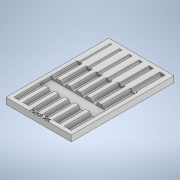
# Autodesk Inventor part: punchTray
Saved by Autodesk Inventor 2020.2 (Build 242310000, 310)
## iProperties
Created: 2019-12-07
Part Number: punchTray
Material: Generic
Document SubType Name: Modeling
Designer: robst
Density: 1 g/cm^3
Appearance: Default
Author: robst
Autodesk Inventor part; units mm, degrees
(part 1 of 2)
ref_plane "YZ Plane" through (0, 0, 0) normal (1, 0, 0) x (0, 1, 0)
ref_plane "XZ Plane" through (0, 0, 0) normal (0, 1, 0) x (-1, 0, 0)
ref_plane "XY Plane" through (0, 0, 0) normal (0, 0, 1) x (1, 0, 0)
sketch "Sketch3" plane through (0, 0, 0) normal (0, 0, 1) x (1, 0, 0)
  line L0 (-52.4636, -4.8895) -> (52.4636, -4.8895)
  line L1 (52.4636, -4.8895) -> (52.4636, 4.8895)
  line L2 (52.4636, 4.8895) -> (-52.4636, 4.8895)
  line L3 (-52.4636, 4.8895) -> (-52.4636, -4.8895)
  line L4 (-52.4636, -4.8895) -> (52.4636, 4.8895) construction
  line L5 (52.4636, -4.8895) -> (-52.4636, 4.8895) construction
  line L6 (46.1136, 4.8895) -> (43.2173, -0.127)
  line L7 (43.2173, -0.127) -> (37.4248, -0.127)
  line L8 (37.4248, -0.127) -> (34.5285, 4.8895)
  line L9 (34.5285, 4.8895) -> (37.4248, 9.906)
  line L10 (37.4248, 9.906) -> (43.2173, 9.906)
  line L11 (43.2173, 9.906) -> (46.1136, 4.8895)
  line L12 (28.1785, 4.8895) -> (25.2822, -0.127)
  line L13 (25.2822, -0.127) -> (19.4897, -0.127)
  line L14 (19.4897, -0.127) -> (16.5934, 4.8895)
  line L15 (16.5934, 4.8895) -> (19.4897, 9.906)
  line L16 (19.4897, 9.906) -> (25.2822, 9.906)
  line L17 (25.2822, 9.906) -> (28.1785, 4.8895)
  line L18 (0, 0) -> (0, 4.8895) construction
  line L19 (10.2434, 4.8895) -> (7.787, 0.635)
  line L20 (7.787, 0.635) -> (2.8744, 0.635)
  line L21 (2.8744, 0.635) -> (0.418, 4.8895)
  line L22 (0.418, 4.8895) -> (2.8744, 9.144)
  line L23 (2.8744, 9.144) -> (7.787, 9.144)
  line L24 (7.787, 9.144) -> (10.2434, 4.8895)
  line L25 (-5.932, 4.8895) -> (-8.3883, 0.635)
  line L26 (-8.3883, 0.635) -> (-13.301, 0.635)
  line L27 (-13.301, 0.635) -> (-15.7573, 4.8895)
  line L28 (-15.7573, 4.8895) -> (-13.301, 9.144)
  line L29 (-13.301, 9.144) -> (-8.3883, 9.144)
  line L30 (-8.3883, 9.144) -> (-5.932, 4.8895)
  line L31 (-22.1073, 4.8895) -> (-24.5416, 0.6731)
  line L32 (-24.5416, 0.6731) -> (-29.4103, 0.6731)
  line L33 (-29.4103, 0.6731) -> (-31.8447, 4.8895)
  line L34 (-31.8447, 4.8895) -> (-29.4103, 9.1059)
  line L35 (-29.4103, 9.1059) -> (-24.5416, 9.1059)
  line L36 (-24.5416, 9.1059) -> (-22.1073, 4.8895)
  line L37 (-38.1947, 4.8895) -> (-40.1744, 1.4605)
  line L38 (-40.1744, 1.4605) -> (-44.1339, 1.4605)
  line L39 (-44.1339, 1.4605) -> (-46.1136, 4.8895)
  line L40 (-46.1136, 4.8895) -> (-44.1339, 8.3185)
  line L41 (-44.1339, 8.3185) -> (-40.1744, 8.3185)
  line L42 (-40.1744, 8.3185) -> (-38.1947, 4.8895)
  point P0 (40.321, 4.8895)
  point P1 (22.3859, 4.8895)
  point P2 (34.5285, 4.8895)
  point P3 (16.5934, 4.8895)
  point P4 (5.3307, 4.8895)
  point P5 (-10.8446, 4.8895)
  point P6 (-26.976, 4.8895)
  point P7 (-42.1541, 4.8895)
  point P8 (0.418, 4.8895)
  point P9 (-15.7573, 4.8895)
  point P10 (-31.8447, 4.8895)
  point P11 (-46.1136, 4.8895)
  dimension "d7" = 10.033
  dimension "d8" = 10.033
  dimension "d13" = 6.35
  dimension "d14" = 6.35
  dimension "d15" = 8.509
  dimension "d16" = 6.35
  dimension "d17" = 8.509
  dimension "d18" = 6.35
  dimension "d19" = 8.4328
  dimension "d20" = 6.35
  dimension "d21" = 6.35
  dimension "d22" = 6.858
  dimension "d23" = 6.35
  dimension "d24" = 4.7625
  constraints: 84 end point, 2 horizontal, 2 midpoint, 1 parallel, 1 perpendicular, 94 other
  measures "d7" distance between parallel lines of L7 L10
  measures "d8" distance between parallel lines of L13 L16
  measures "d13" distance of L6.start L1.end
  measures "d14" distance of L8.end L12.start
  measures "d15" distance between parallel lines of L20 L23
  measures "d16" distance of L14.end L19.start
  measures "d17" distance between parallel lines of L26 L29
  measures "d18" distance of L21.end L25.start
  measures "d19" distance between parallel lines of L32 L35
  measures "d20" distance of L27.end L31.start
  measures "d21" distance of L33.end L37.start
  measures "d22" distance between parallel lines of L38 L41
  measures "d23" distance from line of L39.end L3
  measures "d24" distance between parallel lines of L0 L7
extrude "Extrusion3" add sketch "Sketch3" against normal blind 152.4 contours L3 L2 L39 L38 L37 L33 L32 L31 L27 L26 L25 L21 L20 L19 L14 L13 L12 L8 L7 L6 L1 L0
sketch "Sketch4" plane through (0, 0, 0) normal (0, 0, 1) x (1, 0, 0)
  line L0 (52.4636, -4.8895) -> (-52.4636, -4.8895) projected
  line L1 (52.4636, 4.8895) -> (52.4636, -4.8895) projected
  line L2 (-52.4636, -4.8895) -> (52.4636, -4.8895)
  line L3 (52.4636, -4.8895) -> (52.4636, 4.8895)
  line L4 (52.4636, 4.8895) -> (-52.4636, 4.8895)
  line L5 (-52.4636, 4.8895) -> (-52.4636, -4.8895)
  point P0 (0, 0)
  constraints: 8 end point, 2 parallel, 1 horizontal, 1 perpendicular
extrude "Extrusion4" add sketch "Sketch4" along normal blind 6.35
sketch "Sketch6" plane through (0, 0, -152.4) normal (0, 0, -1) x (-1, 0, 0)
  line L0 (-37.4248, -0.127) -> (-43.2173, -0.127) construction
  line L1 (-40.321, -0.127) -> (-40.321, 4.8895) construction
  line L2 (-52.4636, 4.8895) -> (52.4636, 4.8895) construction
  arc A0 (-44.5438, 4.8895) -> (-36.0983, 4.8895) centre (-40.321, 4.8895) ccw
  line L3 (-34.5285, 4.8895) -> (-37.4248, -0.127)
  line L4 (-37.4248, -0.127) -> (-43.2173, -0.127)
  line L5 (-43.2173, -0.127) -> (-46.1136, 4.8895)
  line L6 (-46.1136, 4.8895) -> (-44.5438, 4.8895)
  line L7 (-34.5285, 4.8895) -> (-36.0983, 4.8895)
  point P0 (0, 0)
  dimension "d31" = 8.4455
  constraints: 12 end point, 3 point on line, 2 coincident, 2 point on circle, 1 centre point, 1 midpoint, 1 vertical, 6 other
  measures "d31" diameter of A0
extrude "5_16_punch" add sketch "Sketch6" against normal blind 46.355
sketch "Sketch7" plane through (0, 0, -152.4) normal (0, 0, -1) x (-1, 0, 0)
  line L0 (-28.1785, 4.8895) -> (-16.5934, 4.8895) projected
  line L1 (-16.5934, 4.8895) -> (-19.4897, -0.127)
  line L2 (-19.4897, -0.127) -> (-25.2822, -0.127)
  line L3 (-25.2822, -0.127) -> (-28.1785, 4.8895)
  arc A0 (-25.8149, 4.8895) -> (-18.9569, 4.8895) centre (-22.3859, 4.8895) ccw
  line L4 (-28.1785, 4.8895) -> (-25.8149, 4.8895)
  line L5 (-10.2434, 4.8895) -> (-16.5934, 4.8895) projected
  line L6 (-16.5934, 4.8895) -> (-18.9569, 4.8895)
  point P0 (0, 0)
  point P1 (-28.1785, 4.8895)
  dimension "d34" = 6.858
  constraints: 10 end point, 2 point on circle, 2 point on line, 1 centre point, 1 coincident, 1 midpoint, 6 other
  measures "d34" diameter of A0
extrude "1_4_punch" add sketch "Sketch7" against normal blind 47.625 contours L0 A0 L1 L2 L3
sketch "Sketch8" plane through (0, 0, -152.4) normal (0, 0, -1) x (-1, 0, 0)
  line L0 (-10.2434, 4.8895) -> (-0.418, 4.8895) projected
  line L1 (-0.418, 4.8895) -> (-2.8744, 0.635)
  line L2 (-2.8744, 0.635) -> (-7.787, 0.635)
  line L3 (-7.787, 0.635) -> (-10.2434, 4.8895)
  arc A0 (-7.966, 4.8895) -> (-2.6955, 4.8895) centre (-5.3307, 4.8895) ccw
  line L4 (-10.2434, 4.8895) -> (-7.787, 0.635) projected
  line L5 (-10.2434, 4.8895) -> (-7.966, 4.8895)
  line L6 (-0.418, 4.8895) -> (-2.6955, 4.8895)
  point P0 (0, 0)
  point P1 (-10.2434, 4.8895)
  dimension "d37" = 5.2705
  constraints: 10 end point, 2 point on circle, 2 point on line, 1 centre point, 1 coincident, 1 midpoint, 6 other
  measures "d37" diameter of A0
extrude "3_16_punch" add sketch "Sketch8" against normal blind 50.8 contours L0 A0 L1 L2 L3
sketch "Sketch9" plane through (0, 0, -152.4) normal (0, 0, -1) x (-1, 0, 0)
  line L0 (13.301, 0.635) -> (8.3883, 0.635) construction
  line L1 (10.8446, 0.635) -> (10.8446, 4.8895) construction
  line L2 (-52.4636, 4.8895) -> (52.4636, 4.8895) construction
  line L3 (15.7573, 4.8895) -> (13.301, 0.635) projected
  line L4 (15.7573, 4.8895) -> (13.301, 0.635)
  line L5 (13.301, 0.635) -> (8.3883, 0.635)
  line L6 (8.3883, 0.635) -> (5.932, 4.8895)
  arc A0 (8.6063, 4.8895) -> (13.083, 4.8895) centre (10.8446, 4.8895) ccw
  line L7 (8.3883, 0.635) -> (5.932, 4.8895) projected
  line L8 (5.932, 4.8895) -> (8.6063, 4.8895)
  line L9 (22.1073, 4.8895) -> (15.7573, 4.8895) projected
  line L10 (15.7573, 4.8895) -> (13.083, 4.8895)
  point P0 (0, 0)
  point P1 (13.301, 0.635)
  dimension "d40" = 4.4768
  constraints: 12 end point, 3 point on line, 2 coincident, 2 point on circle, 1 centre point, 1 midpoint, 1 vertical, 6 other
  measures "d40" diameter of A0
extrude "5_32_punch" add sketch "Sketch9" against normal blind 50.8
sketch "Sketch11" plane through (0, 0, -152.4) normal (0, 0, -1) x (-1, 0, 0)
  line L0 (22.1073, 4.8895) -> (31.8447, 4.8895) projected
  line L1 (29.4103, 0.6731) -> (31.8447, 4.8895) projected
  line L2 (31.8447, 4.8895) -> (29.4103, 0.6731)
  line L3 (29.4103, 0.6731) -> (24.5416, 0.6731)
  line L4 (24.5416, 0.6731) -> (22.1073, 4.8895)
  arc A0 (25.1345, 4.8895) -> (28.8175, 4.8895) centre (26.976, 4.8895) ccw
  line L5 (22.1073, 4.8895) -> (24.5416, 0.6731) projected
  line L6 (22.1073, 4.8895) -> (25.1345, 4.8895)
  line L7 (31.8447, 4.8895) -> (28.8175, 4.8895)
  point P0 (0, 0)
  point P1 (29.4103, 0.6731)
  dimension "d44" = 3.683
  constraints: 10 end point, 2 point on circle, 2 point on line, 1 centre point, 1 coincident, 1 midpoint, 6 other
  measures "d44" diameter of A0
extrude "1_8_punch" add sketch "Sketch11" against normal blind 50.8 contours L0 A0 L1 L3 L4
sketch "Sketch12" plane through (0, 0, -152.4) normal (0, 0, -1) x (-1, 0, 0)
  line L0 (40.1744, 1.4605) -> (44.1339, 1.4605) construction
  line L1 (42.1541, 1.4605) -> (42.1541, 4.8895) construction
  line L2 (-52.4636, 4.8895) -> (52.4636, 4.8895) construction
  line L3 (44.1339, 1.4605) -> (46.1136, 4.8895) projected
  line L4 (46.1136, 4.8895) -> (44.1339, 1.4605)
  line L5 (44.1339, 1.4605) -> (40.1744, 1.4605)
  line L6 (40.1744, 1.4605) -> (38.1947, 4.8895)
  arc A0 (41.1064, 4.8895) -> (43.2019, 4.8895) centre (42.1541, 4.8895) ccw
  line L7 (38.1947, 4.8895) -> (28.8175, 4.8895) projected
  line L8 (38.1947, 4.8895) -> (41.1064, 4.8895)
  line L9 (46.1136, 4.8895) -> (43.2019, 4.8895)
  point P0 (0, 0)
  point P1 (44.1339, 1.4605)
  dimension "d47" = 2.0955
  constraints: 12 end point, 3 point on line, 2 coincident, 2 point on circle, 1 centre point, 1 midpoint, 1 vertical, 6 other
  measures "d47" diameter of A0
extrude "1_16_punch" add sketch "Sketch12" against normal blind 50.8
sketch "Sketch5" plane through (0, 0, -152.4) normal (0, 0, -1) x (-1, 0, 0)
  line L0 (-52.4636, 4.8895) -> (-52.4636, -4.8895) projected
  line L1 (52.4636, 4.8895) -> (46.1136, 4.8895) projected
  line L2 (-52.4636, -4.8895) -> (52.4636, -4.8895)
  line L3 (52.4636, -4.8895) -> (52.4636, 4.8895)
  line L4 (52.4636, 4.8895) -> (-52.4636, 4.8895)
  line L5 (-52.4636, 4.8895) -> (-52.4636, -4.8895)
  point P0 (0, 0)
  point P1 (-52.4636, 4.8895)
  constraints: 8 end point, 2 parallel, 1 horizontal, 1 perpendicular
extrude "Extrusion5" add sketch "Sketch5" along normal blind 6.35
sketch "Sketch13" plane through (-52.4636, 4.8895, 6.35) normal (0, 1, 0) x (1, 0, 0)
  line L0 (6.35, 6.35) -> (6.35, 107.95) projected
  line L1 (98.5772, 6.35) -> (98.5772, 112.395) projected
  line L2 (6.35, 47.625) -> (98.5772, 47.625)
  line L3 (98.5772, 47.625) -> (98.5772, 66.675)
  line L4 (98.5772, 66.675) -> (6.35, 66.675)
  line L5 (6.35, 66.675) -> (6.35, 47.625)
  line L6 (6.35, 57.15) -> (98.5772, 57.15) construction
  line L7 (14.2689, 6.35) -> (6.35, 6.35) construction
  point P0 (52.4636, 6.35)
  point P1 (6.35, 66.675)
  dimension "d50" = 19.05
  dimension "d51" = 50.8
  constraints: 10 end point, 2 midpoint, 2 parallel, 2 point on line, 1 horizontal, 1 perpendicular
  measures "d50" distance between parallel lines of L4 L2
  measures "d51" distance between parallel lines of L6 L7
extrude "Extrusion12" cut sketch "Sketch13" against normal blind 5.08
sketch "Sketch14" plane through (-52.4636, 4.8895, 6.35) normal (0, 1, 0) x (1, 0, 0)
  line L0 (0, 165.1) -> (0, 0) construction
  line L1 (0, 3.175) -> (104.9272, 3.175) construction
  line L2 (0, 0) -> (104.9272, 0) construction
  spline S0 degree 2 poles (40.766, 4.1836) (40.766, 3.8543) (40.5314, 3.2615) (40.3214, 3.0556) knots 0 0 0 1 2 2 2
  spline S1 degree 2 poles (40.3214, 3.0556) (40.0579, 2.7963) (39.3458, 2.5287) (38.8024, 2.5287) knots 0 0 0 1 2 2 2
  line L3 (38.8024, 2.5287) -> (38.2301, 2.5287)
  line L4 (38.2301, 2.5287) -> (38.2301, 0.635)
  line L5 (38.2301, 0.635) -> (37.555, 0.635)
  line L6 (37.555, 0.635) -> (37.555, 5.715)
  line L7 (37.555, 5.715) -> (38.8312, 5.715)
  spline S2 degree 2 poles (38.8312, 5.715) (39.284, 5.715) (39.918, 5.5668) (40.1609, 5.398) knots 0 0 0 1 2 2 2
  spline S3 degree 2 poles (40.1609, 5.398) (40.4449, 5.2045) (40.766, 4.6076) (40.766, 4.1836) knots 0 0 0 1 2 2 2
  spline S4 degree 2 poles (40.0621, 4.163) (40.0621, 4.4265) (39.8809, 4.8134) (39.6957, 4.9369) knots 0 0 0 1 2 2 2
  spline S5 degree 2 poles (39.6957, 4.9369) (39.5351, 5.044) (39.107, 5.1304) (38.79, 5.1304) knots 0 0 0 1 2 2 2
  line L8 (38.79, 5.1304) -> (38.2301, 5.1304)
  line L9 (38.2301, 5.1304) -> (38.2301, 3.105)
  line L10 (38.2301, 3.105) -> (38.6912, 3.105)
  spline S6 degree 2 poles (38.6912, 3.105) (39.1029, 3.105) (39.6092, 3.2368) (39.7739, 3.4097) knots 0 0 0 1 2 2 2
  spline S7 degree 2 poles (39.7739, 3.4097) (39.9262, 3.562) (40.0621, 3.9201) (40.0621, 4.163) knots 0 0 0 1 2 2 2
  line L11 (44.3228, 0.635) -> (43.6806, 0.635)
  line L12 (43.6806, 0.635) -> (43.6806, 1.0549)
  spline S8 degree 2 poles (43.6806, 1.0549) (43.3842, 0.7956) (42.8532, 0.528) (42.5238, 0.528) knots 0 0 0 1 2 2 2
  spline S9 degree 2 poles (42.5238, 0.528) (42.2768, 0.528) (41.8364, 0.6926) (41.6758, 0.8697) knots 0 0 0 1 2 2 2
  spline S10 degree 2 poles (41.6758, 0.8697) (41.5111, 1.0467) (41.33, 1.586) (41.33, 1.9729) knots 0 0 0 1 2 2 2
  line L13 (41.33, 1.9729) -> (41.33, 4.4471)
  line L14 (41.33, 4.4471) -> (41.9722, 4.4471)
  line L15 (41.9722, 4.4471) -> (41.9722, 2.2734)
  spline S11 degree 2 poles (41.9722, 2.2734) (41.9722, 1.9688) (42.0175, 1.5695) (42.0957, 1.4213) knots 0 0 0 1 2 2 2
  spline S12 degree 2 poles (42.0957, 1.4213) (42.1739, 1.2731) (42.4415, 1.1372) (42.6926, 1.1372) knots 0 0 0 1 2 2 2
  spline S13 degree 2 poles (42.6926, 1.1372) (42.9273, 1.1372) (43.4583, 1.4048) (43.6806, 1.5983) knots 0 0 0 1 2 2 2
  line L16 (43.6806, 1.5983) -> (43.6806, 4.4471)
  line L17 (43.6806, 4.4471) -> (44.3228, 4.4471)
  line L18 (44.3228, 4.4471) -> (44.3228, 0.635)
  line L19 (48.2461, 0.635) -> (47.6038, 0.635)
  line L20 (47.6038, 0.635) -> (47.6038, 2.8086)
  spline S14 degree 2 poles (47.6038, 2.8086) (47.6038, 3.0721) (47.5544, 3.5249) (47.4803, 3.6608) knots 0 0 0 1 2 2 2
  spline S15 degree 2 poles (47.4803, 3.6608) (47.4021, 3.8049) (47.1222, 3.9448) (46.8834, 3.9448) knots 0 0 0 1 2 2 2
  spline S16 degree 2 poles (46.8834, 3.9448) (46.6447, 3.9448) (46.1383, 3.6896) (45.8954, 3.4838) knots 0 0 0 1 2 2 2
  line L21 (45.8954, 3.4838) -> (45.8954, 0.635)
  line L22 (45.8954, 0.635) -> (45.2532, 0.635)
  line L23 (45.2532, 0.635) -> (45.2532, 4.4471)
  line L24 (45.2532, 4.4471) -> (45.8954, 4.4471)
  line L25 (45.8954, 4.4471) -> (45.8954, 4.023)
  spline S17 degree 2 poles (45.8954, 4.023) (46.1836, 4.2824) (46.7393, 4.5541) (47.0522, 4.5541) knots 0 0 0 1 2 2 2
  spline S18 degree 2 poles (47.0522, 4.5541) (47.6121, 4.5541) (48.2461, 3.8131) (48.2461, 3.1091) knots 0 0 0 1 2 2 2
  line L26 (48.2461, 3.1091) -> (48.2461, 0.635)
  spline S19 degree 2 poles (50.6626, 0.5485) (50.2673, 0.5485) (49.6128, 0.7914) (49.3781, 1.0384) knots 0 0 0 1 2 2 2
  spline S20 degree 2 poles (49.3781, 1.0384) (49.1435, 1.2813) (48.8841, 2.0306) (48.8841, 2.5328) knots 0 0 0 1 2 2 2
  spline S21 degree 2 poles (48.8841, 2.5328) (48.8841, 3.035) (49.1517, 3.7678) (49.3781, 4.0148) knots 0 0 0 1 2 2 2
  spline S22 degree 2 poles (49.3781, 4.0148) (49.6046, 4.2659) (50.2756, 4.5335) (50.6626, 4.5335) knots 0 0 0 1 2 2 2
  spline S23 degree 2 poles (50.6626, 4.5335) (50.9754, 4.5335) (51.56, 4.3565) (51.7864, 4.2412) knots 0 0 0 1 2 2 2
  line L27 (51.7864, 4.2412) -> (51.7864, 3.5208)
  line L28 (51.7864, 3.5208) -> (51.7494, 3.5208)
  spline S24 degree 2 poles (51.7494, 3.5208) (51.6794, 3.5784) (51.4653, 3.7266) (51.313, 3.8049) knots 0 0 0 1 2 2 2
  spline S25 degree 2 poles (51.313, 3.8049) (51.1771, 3.8707) (50.8149, 3.9736) (50.6502, 3.9736) knots 0 0 0 1 2 2 2
  spline S26 degree 2 poles (50.6502, 3.9736) (50.1521, 3.9736) (49.5469, 3.2203) (49.5469, 2.5328) knots 0 0 0 1 2 2 2
  spline S27 degree 2 poles (49.5469, 2.5328) (49.5469, 1.8618) (50.1315, 1.1084) (50.6502, 1.1084) knots 0 0 0 1 2 2 2
  spline S28 degree 2 poles (50.6502, 1.1084) (50.9631, 1.1084) (51.5312, 1.3678) (51.7494, 1.5695) knots 0 0 0 1 2 2 2
  line L29 (51.7494, 1.5695) -> (51.7864, 1.5695)
  line L30 (51.7864, 1.5695) -> (51.7864, 0.8491)
  spline S29 degree 2 poles (51.7864, 0.8491) (51.6917, 0.8038) (51.4036, 0.6762) (51.2883, 0.6474) knots 0 0 0 1 2 2 2
  spline S30 degree 2 poles (51.2883, 0.6474) (51.1236, 0.5979) (50.8643, 0.5485) (50.6626, 0.5485) knots 0 0 0 1 2 2 2
  line L31 (55.3638, 0.635) -> (54.7216, 0.635)
  line L32 (54.7216, 0.635) -> (54.7216, 2.8086)
  spline S31 degree 2 poles (54.7216, 2.8086) (54.7216, 3.0721) (54.6722, 3.5249) (54.5981, 3.6608) knots 0 0 0 1 2 2 2
  spline S32 degree 2 poles (54.5981, 3.6608) (54.5199, 3.8049) (54.24, 3.9448) (54.0012, 3.9448) knots 0 0 0 1 2 2 2
  spline S33 degree 2 poles (54.0012, 3.9448) (53.7624, 3.9448) (53.2561, 3.6896) (53.0132, 3.4838) knots 0 0 0 1 2 2 2
  line L33 (53.0132, 3.4838) -> (53.0132, 0.635)
  line L34 (53.0132, 0.635) -> (52.371, 0.635)
  line L35 (52.371, 0.635) -> (52.371, 5.9414)
  line L36 (52.371, 5.9414) -> (53.0132, 5.9414)
  line L37 (53.0132, 5.9414) -> (53.0132, 4.023)
  spline S34 degree 2 poles (53.0132, 4.023) (53.3014, 4.2824) (53.8571, 4.5541) (54.17, 4.5541) knots 0 0 0 1 2 2 2
  spline S35 degree 2 poles (54.17, 4.5541) (54.7298, 4.5541) (55.3638, 3.8131) (55.3638, 3.1091) knots 0 0 0 1 2 2 2
  line L38 (55.3638, 3.1091) -> (55.3638, 0.635)
  spline S36 degree 2 poles (59.9128, 0.5444) (59.3611, 0.5444) (58.5872, 0.775) (58.2455, 0.9396) knots 0 0 0 1 2 2 2
  line L39 (58.2455, 0.9396) -> (58.2455, 1.7877)
  line L40 (58.2455, 1.7877) -> (58.2949, 1.7877)
  spline S37 degree 2 poles (58.2949, 1.7877) (58.6284, 1.4748) (59.4723, 1.129) (59.8634, 1.129) knots 0 0 0 1 2 2 2
  spline S38 degree 2 poles (59.8634, 1.129) (60.4232, 1.129) (60.9955, 1.5942) (60.9955, 1.977) knots 0 0 0 1 2 2 2
  spline S39 degree 2 poles (60.9955, 1.977) (60.9955, 2.2817) (60.6949, 2.6604) (60.3697, 2.7551) knots 0 0 0 1 2 2 2
  spline S40 degree 2 poles (60.3697, 2.7551) (60.1351, 2.821) (59.744, 2.9115) (59.4517, 2.9856) knots 0 0 0 1 2 2 2
  spline S41 degree 2 poles (59.4517, 2.9856) (59.1882, 3.0556) (58.7724, 3.2656) (58.6119, 3.4344) knots 0 0 0 1 2 2 2
  spline S42 degree 2 poles (58.6119, 3.4344) (58.4555, 3.6031) (58.2826, 4.056) (58.2826, 4.3524) knots 0 0 0 1 2 2 2
  spline S43 degree 2 poles (58.2826, 4.3524) (58.2826, 4.9699) (59.2459, 5.8056) (59.991, 5.8056) knots 0 0 0 1 2 2 2
  spline S44 degree 2 poles (59.991, 5.8056) (60.4191, 5.8056) (61.1766, 5.6368) (61.5018, 5.4762) knots 0 0 0 1 2 2 2
  line L41 (61.5018, 5.4762) -> (61.5018, 4.6694)
  line L42 (61.5018, 4.6694) -> (61.4524, 4.6694)
  spline S45 degree 2 poles (61.4524, 4.6694) (61.2095, 4.8917) (60.452, 5.221) (60.0363, 5.221) knots 0 0 0 1 2 2 2
  spline S46 degree 2 poles (60.0363, 5.221) (59.567, 5.221) (58.9865, 4.7805) (58.9865, 4.4224) knots 0 0 0 1 2 2 2
  spline S47 degree 2 poles (58.9865, 4.4224) (58.9865, 4.1013) (59.3282, 3.7184) (59.6493, 3.632) knots 0 0 0 1 2 2 2
  spline S48 degree 2 poles (59.6493, 3.632) (59.8634, 3.5743) (60.485, 3.4261) (60.6908, 3.3644) knots 0 0 0 1 2 2 2
  spline S49 degree 2 poles (60.6908, 3.3644) (61.2136, 3.2038) (61.6994, 2.5575) (61.6994, 2.0841) knots 0 0 0 1 2 2 2
  spline S50 degree 2 poles (61.6994, 2.0841) (61.6994, 1.7836) (61.4565, 1.2072) (61.2383, 1.0055) knots 0 0 0 1 2 2 2
  spline S51 degree 2 poles (61.2383, 1.0055) (60.9955, 0.7832) (60.3779, 0.5444) (59.9128, 0.5444) knots 0 0 0 1 2 2 2
  spline S52 degree 2 poles (63.9924, 0.5485) (63.0785, 0.5485) (62.074, 1.5736) (62.074, 2.5204) knots 0 0 0 1 2 2 2
  spline S53 degree 2 poles (62.074, 2.5204) (62.074, 3.4508) (63.0497, 4.5541) (63.836, 4.5541) knots 0 0 0 1 2 2 2
  spline S54 degree 2 poles (63.836, 4.5541) (64.19, 4.5541) (64.7375, 4.3483) (64.9392, 4.1301) knots 0 0 0 1 2 2 2
  spline S55 degree 2 poles (64.9392, 4.1301) (65.1451, 3.9119) (65.3633, 3.282) (65.3633, 2.8251) knots 0 0 0 1 2 2 2
  line L43 (65.3633, 2.8251) -> (65.3633, 2.4752)
  line L44 (65.3633, 2.4752) -> (62.7245, 2.4752)
  spline S56 degree 2 poles (62.7245, 2.4752) (62.7245, 1.8124) (63.3914, 1.1084) (63.9842, 1.1084) knots 0 0 0 1 2 2 2
  spline S57 degree 2 poles (63.9842, 1.1084) (64.1941, 1.1084) (64.6017, 1.2031) (64.7663, 1.2772) knots 0 0 0 1 2 2 2
  spline S58 degree 2 poles (64.7663, 1.2772) (64.9392, 1.3595) (65.178, 1.5036) (65.2562, 1.5695) knots 0 0 0 1 2 2 2
  line L45 (65.2562, 1.5695) -> (65.2933, 1.5695)
  line L46 (65.2933, 1.5695) -> (65.2933, 0.8697)
  spline S59 degree 2 poles (65.2933, 0.8697) (65.1821, 0.8244) (64.8446, 0.6926) (64.7128, 0.6556) knots 0 0 0 1 2 2 2
  spline S60 degree 2 poles (64.7128, 0.6556) (64.5276, 0.6021) (64.2229, 0.5485) (63.9924, 0.5485) knots 0 0 0 1 2 2 2
  spline S61 degree 2 poles (64.7375, 2.965) (64.7293, 3.2244) (64.6223, 3.6031) (64.5193, 3.7308) knots 0 0 0 1 2 2 2
  spline S62 degree 2 poles (64.5193, 3.7308) (64.4082, 3.8748) (64.0583, 4.0272) (63.7989, 4.0272) knots 0 0 0 1 2 2 2
  spline S63 degree 2 poles (63.7989, 4.0272) (63.5437, 4.0272) (63.1855, 3.8748) (63.0373, 3.7266) knots 0 0 0 1 2 2 2
  spline S64 degree 2 poles (63.0373, 3.7266) (62.8932, 3.5743) (62.745, 3.2079) (62.7245, 2.965) knots 0 0 0 1 2 2 2
  line L47 (62.7245, 2.965) -> (64.7375, 2.965)
  spline S65 degree 2 poles (67.1664, 0.5609) (66.6436, 0.5609) (66.0549, 1.1578) (66.0549, 1.8041) knots 0 0 0 1 2 2 2
  line L48 (66.0549, 1.8041) -> (66.0549, 3.916)
  line L49 (66.0549, 3.916) -> (65.6226, 3.916)
  line L50 (65.6226, 3.916) -> (65.6226, 4.4471)
  line L51 (65.6226, 4.4471) -> (66.0549, 4.4471)
  line L52 (66.0549, 4.4471) -> (66.0549, 5.5421)
  line L53 (66.0549, 5.5421) -> (66.6971, 5.5421)
  line L54 (66.6971, 5.5421) -> (66.6971, 4.4471)
  line L55 (66.6971, 4.4471) -> (67.8786, 4.4471)
  line L56 (67.8786, 4.4471) -> (67.8786, 3.916)
  line L57 (67.8786, 3.916) -> (66.6971, 3.916)
  line L58 (66.6971, 3.916) -> (66.6971, 2.1005)
  spline S66 degree 2 poles (66.6971, 2.1005) (66.6971, 1.8124) (66.7177, 1.4954) (66.7876, 1.3595) knots 0 0 0 1 2 2 2
  spline S67 degree 2 poles (66.7876, 1.3595) (66.8453, 1.2402) (67.1046, 1.1208) (67.3269, 1.1208) knots 0 0 0 1 2 2 2
  spline S68 degree 2 poles (67.3269, 1.1208) (67.4834, 1.1208) (67.7756, 1.2155) (67.8415, 1.2443) knots 0 0 0 1 2 2 2
  line L59 (67.8415, 1.2443) -> (67.8786, 1.2443)
  line L60 (67.8786, 1.2443) -> (67.8786, 0.6679)
  spline S69 degree 2 poles (67.8786, 0.6679) (67.6974, 0.6185) (67.3269, 0.5609) (67.1664, 0.5609) knots 0 0 0 1 2 2 2
  point P0 (52.4636, 6.35)
  dimension "d54" = 3.175
  constraints: 2 end point, 1 horizontal, 1 parallel, 1 point on line
  measures "d54" distance between parallel lines of L1 L2
extrude "Extrusion13" cut sketch "Sketch14" against normal blind 3.175
sketch "Sketch15" plane through (-52.4636, -4.8895, 6.35) normal (0, -1, 0) x (1, 0, 0)
  line L0 (104.9272, -165.1) -> (104.9272, 0) construction
  line L1 (104.9272, -82.55) -> (0, -82.55) construction
  line L2 (0, -165.1) -> (0, 0) construction
  spline S0 degree 2 poles (70.5282, -95.2449) (70.5282, -94.3752) (71.2332, -92.9755) (71.8249, -92.5844) knots 0 0 0 1 2 2 2
  spline S1 degree 2 poles (71.8249, -92.5844) (72.3086, -92.2808) (73.3018, -92.075) (74.0737, -92.075) knots 0 0 0 1 2 2 2
  line L3 (74.0737, -92.075) -> (75.5351, -92.075)
  line L4 (75.5351, -92.075) -> (75.5351, -98.425)
  line L5 (75.5351, -98.425) -> (74.0891, -98.425)
  spline S2 degree 2 poles (74.0891, -98.425) (73.1937, -98.425) (72.1748, -98.1574) (71.8146, -97.9207) knots 0 0 0 1 2 2 2
  spline S3 degree 2 poles (71.8146, -97.9207) (71.2023, -97.5142) (70.5282, -96.1711) (70.5282, -95.2449) knots 0 0 0 1 2 2 2
  spline S4 degree 2 poles (71.4081, -95.2551) (71.4081, -95.9859) (71.8918, -97.0202) (72.3704, -97.3135) knots 0 0 0 1 2 2 2
  spline S5 degree 2 poles (72.3704, -97.3135) (72.71, -97.5142) (73.4768, -97.6943) (74.0479, -97.6943) knots 0 0 0 1 2 2 2
  line L6 (74.0479, -97.6943) -> (74.6912, -97.6943)
  line L7 (74.6912, -97.6943) -> (74.6912, -92.8057)
  line L8 (74.6912, -92.8057) -> (74.0479, -92.8057)
  spline S6 degree 2 poles (74.0479, -92.8057) (73.487, -92.8057) (72.638, -92.9858) (72.2932, -93.2277) knots 0 0 0 1 2 2 2
  spline S7 degree 2 poles (72.2932, -93.2277) (71.8507, -93.5261) (71.4081, -94.5141) (71.4081, -95.2551) knots 0 0 0 1 2 2 2
  spline S8 degree 2 poles (67.6053, -91.9669) (68.7477, -91.9669) (70.0033, -93.2483) (70.0033, -94.4318) knots 0 0 0 1 2 2 2
  spline S9 degree 2 poles (70.0033, -94.4318) (70.0033, -95.5948) (68.7837, -96.9739) (67.8009, -96.9739) knots 0 0 0 1 2 2 2
  spline S10 degree 2 poles (67.8009, -96.9739) (67.3583, -96.9739) (66.6739, -96.7166) (66.4218, -96.4438) knots 0 0 0 1 2 2 2
  spline S11 degree 2 poles (66.4218, -96.4438) (66.1645, -96.1711) (65.8917, -95.3838) (65.8917, -94.8126) knots 0 0 0 1 2 2 2
  line L9 (65.8917, -94.8126) -> (65.8917, -94.3752)
  line L10 (65.8917, -94.3752) -> (69.1902, -94.3752)
  spline S12 degree 2 poles (69.1902, -94.3752) (69.1902, -93.5467) (68.3566, -92.6668) (67.6156, -92.6668) knots 0 0 0 1 2 2 2
  spline S13 degree 2 poles (67.6156, -92.6668) (67.3532, -92.6668) (66.8437, -92.7851) (66.6379, -92.8778) knots 0 0 0 1 2 2 2
  spline S14 degree 2 poles (66.6379, -92.8778) (66.4218, -92.9807) (66.1233, -93.1608) (66.0255, -93.2431) knots 0 0 0 1 2 2 2
  line L11 (66.0255, -93.2431) -> (65.9792, -93.2431)
  line L12 (65.9792, -93.2431) -> (65.9792, -92.3683)
  spline S15 degree 2 poles (65.9792, -92.3683) (66.1182, -92.3117) (66.5401, -92.147) (66.7048, -92.1007) knots 0 0 0 1 2 2 2
  spline S16 degree 2 poles (66.7048, -92.1007) (66.9364, -92.0338) (67.3172, -91.9669) (67.6053, -91.9669) knots 0 0 0 1 2 2 2
  spline S17 degree 2 poles (66.6739, -94.9876) (66.6842, -95.3118) (66.818, -95.7852) (66.9466, -95.9447) knots 0 0 0 1 2 2 2
  spline S18 degree 2 poles (66.9466, -95.9447) (67.0856, -96.1248) (67.523, -96.3152) (67.8472, -96.3152) knots 0 0 0 1 2 2 2
  spline S19 degree 2 poles (67.8472, -96.3152) (68.1662, -96.3152) (68.6139, -96.1248) (68.7992, -95.9395) knots 0 0 0 1 2 2 2
  spline S20 degree 2 poles (68.7992, -95.9395) (68.9793, -95.7491) (69.1645, -95.2912) (69.1902, -94.9876) knots 0 0 0 1 2 2 2
  line L13 (69.1902, -94.9876) -> (66.6739, -94.9876)
  spline S21 degree 2 poles (63.7922, -91.9618) (64.2708, -91.9618) (65.0993, -92.2191) (65.372, -92.3632) knots 0 0 0 1 2 2 2
  line L14 (65.372, -92.3632) -> (65.372, -93.2637)
  line L15 (65.372, -93.2637) -> (65.3308, -93.2637)
  spline S22 degree 2 poles (65.3308, -93.2637) (65.2279, -93.1814) (64.9501, -92.9858) (64.7185, -92.8778) knots 0 0 0 1 2 2 2
  spline S23 degree 2 poles (64.7185, -92.8778) (64.5178, -92.78) (64.0238, -92.6359) (63.7614, -92.6359) knots 0 0 0 1 2 2 2
  spline S24 degree 2 poles (63.7614, -92.6359) (63.571, -92.6359) (63.1336, -92.7234) (63.0306, -92.7954) knots 0 0 0 1 2 2 2
  spline S25 degree 2 poles (63.0306, -92.7954) (62.8814, -92.8932) (62.7476, -93.1145) (62.7476, -93.3409) knots 0 0 0 1 2 2 2
  spline S26 degree 2 poles (62.7476, -93.3409) (62.7476, -93.6239) (63.0564, -93.9172) (63.4526, -94.015) knots 0 0 0 1 2 2 2
  spline S27 degree 2 poles (63.4526, -94.015) (63.607, -94.051) (64.101, -94.1539) (64.312, -94.2105) knots 0 0 0 1 2 2 2
  spline S28 degree 2 poles (64.312, -94.2105) (64.8574, -94.3701) (65.3514, -95.0287) (65.3514, -95.497) knots 0 0 0 1 2 2 2
  spline S29 degree 2 poles (65.3514, -95.497) (65.3514, -96.1454) (64.3789, -96.9533) (63.5761, -96.9533) knots 0 0 0 1 2 2 2
  spline S30 degree 2 poles (63.5761, -96.9533) (63.1799, -96.9533) (62.3771, -96.7577) (62.1044, -96.6085) knots 0 0 0 1 2 2 2
  line L16 (62.1044, -96.6085) -> (62.1044, -95.7491)
  line L17 (62.1044, -95.7491) -> (62.1456, -95.7491)
  spline S31 degree 2 poles (62.1456, -95.7491) (62.4543, -95.9962) (63.2056, -96.2792) (63.5915, -96.2792) knots 0 0 0 1 2 2 2
  spline S32 degree 2 poles (63.5915, -96.2792) (63.9878, -96.2792) (64.5332, -95.9447) (64.5332, -95.6102) knots 0 0 0 1 2 2 2
  spline S33 degree 2 poles (64.5332, -95.6102) (64.5332, -95.3066) (64.209, -95.0133) (63.8488, -94.9207) knots 0 0 0 1 2 2 2
  spline S34 degree 2 poles (63.8488, -94.9207) (63.6739, -94.8744) (63.2313, -94.7817) (62.9895, -94.7251) knots 0 0 0 1 2 2 2
  spline S35 degree 2 poles (62.9895, -94.7251) (62.4646, -94.5913) (61.9294, -93.979) (61.9294, -93.4489) knots 0 0 0 1 2 2 2
  spline S36 degree 2 poles (61.9294, -93.4489) (61.9294, -93.1402) (62.1713, -92.5947) (62.408, -92.394) knots 0 0 0 1 2 2 2
  spline S37 degree 2 poles (62.408, -92.394) (62.6601, -92.1831) (63.3034, -91.9618) (63.7922, -91.9618) knots 0 0 0 1 2 2 2
  line L18 (60.3651, -92.075) -> (61.1678, -92.075)
  line L19 (61.1678, -92.075) -> (61.1678, -96.8401)
  line L20 (61.1678, -96.8401) -> (60.3651, -96.8401)
  line L21 (60.3651, -96.8401) -> (60.3651, -92.075)
  line L22 (60.3085, -97.6325) -> (61.2193, -97.6325)
  line L23 (61.2193, -97.6325) -> (61.2193, -98.4662)
  line L24 (61.2193, -98.4662) -> (60.3085, -98.4662)
  line L25 (60.3085, -98.4662) -> (60.3085, -97.6325)
  spline S38 degree 2 poles (59.0169, -91.3134) (58.9345, -91.2774) (58.6206, -91.1642) (58.4199, -91.1179) knots 0 0 0 1 2 2 2
  spline S39 degree 2 poles (58.4199, -91.1179) (58.1987, -91.0613) (57.823, -90.9944) (57.6018, -90.9944) knots 0 0 0 1 2 2 2
  spline S40 degree 2 poles (57.6018, -90.9944) (57.2313, -90.9944) (56.7167, -91.1899) (56.5726, -91.3649) knots 0 0 0 1 2 2 2
  spline S41 degree 2 poles (56.5726, -91.3649) (56.4336, -91.5398) (56.3256, -91.9978) (56.3256, -92.2911) knots 0 0 0 1 2 2 2
  line L26 (56.3256, -92.2911) -> (56.3256, -92.7079)
  spline S42 degree 2 poles (56.3256, -92.7079) (56.6498, -92.4249) (57.2724, -92.1573) (57.7407, -92.1573) knots 0 0 0 1 2 2 2
  spline S43 degree 2 poles (57.7407, -92.1573) (58.5537, -92.1573) (59.516, -93.3666) (59.516, -94.5038) knots 0 0 0 1 2 2 2
  spline S44 degree 2 poles (59.516, -94.5038) (59.516, -95.0956) (59.1815, -96.0116) (58.9037, -96.3358) knots 0 0 0 1 2 2 2
  spline S45 degree 2 poles (58.9037, -96.3358) (58.6361, -96.6394) (57.9002, -96.9739) (57.5091, -96.9739) knots 0 0 0 1 2 2 2
  spline S46 degree 2 poles (57.5091, -96.9739) (57.1386, -96.9739) (56.5983, -96.7989) (56.3256, -96.6394) knots 0 0 0 1 2 2 2
  line L27 (56.3256, -96.6394) -> (56.2793, -96.8401)
  line L28 (56.2793, -96.8401) -> (55.5228, -96.8401)
  line L29 (55.5228, -96.8401) -> (55.5228, -92.6205)
  spline S47 degree 2 poles (55.5228, -92.6205) (55.5228, -91.406) (56.5777, -90.2739) (57.6635, -90.2739) knots 0 0 0 1 2 2 2
  spline S48 degree 2 poles (57.6635, -90.2739) (58.0134, -90.2739) (58.7441, -90.3872) (59.058, -90.4798) knots 0 0 0 1 2 2 2
  line L30 (59.058, -90.4798) -> (59.058, -91.3134)
  line L31 (59.058, -91.3134) -> (59.0169, -91.3134)
  line L32 (56.3256, -93.3666) -> (56.3256, -95.9859)
  spline S49 degree 2 poles (56.3256, -95.9859) (56.624, -96.1299) (57.1283, -96.2534) (57.3805, -96.2534) knots 0 0 0 1 2 2 2
  spline S50 degree 2 poles (57.3805, -96.2534) (57.9877, -96.2534) (58.6875, -95.3581) (58.6875, -94.5193) knots 0 0 0 1 2 2 2
  spline S51 degree 2 poles (58.6875, -94.5193) (58.6875, -93.7268) (58.1575, -92.8983) (57.5606, -92.8983) knots 0 0 0 1 2 2 2
  spline S52 degree 2 poles (57.5606, -92.8983) (57.2467, -92.8983) (56.588, -93.1453) (56.3256, -93.3666) knots 0 0 0 1 2 2 2
  line L33 (50.6188, -92.075) -> (51.4216, -92.075)
  line L34 (51.4216, -92.075) -> (51.4216, -94.792)
  spline S53 degree 2 poles (51.4216, -94.792) (51.4216, -95.1214) (51.4833, -95.6874) (51.5759, -95.8572) knots 0 0 0 1 2 2 2
  spline S54 degree 2 poles (51.5759, -95.8572) (51.6737, -96.0373) (52.0236, -96.2123) (52.3221, -96.2123) knots 0 0 0 1 2 2 2
  spline S55 degree 2 poles (52.3221, -96.2123) (52.6206, -96.2123) (53.2535, -95.8932) (53.5571, -95.6359) knots 0 0 0 1 2 2 2
  line L35 (53.5571, -95.6359) -> (53.5571, -92.075)
  line L36 (53.5571, -92.075) -> (54.3599, -92.075)
  line L37 (54.3599, -92.075) -> (54.3599, -96.8401)
  line L38 (54.3599, -96.8401) -> (53.5571, -96.8401)
  line L39 (53.5571, -96.8401) -> (53.5571, -96.31)
  spline S56 degree 2 poles (53.5571, -96.31) (53.1969, -96.6342) (52.5022, -96.9739) (52.1111, -96.9739) knots 0 0 0 1 2 2 2
  spline S57 degree 2 poles (52.1111, -96.9739) (51.4113, -96.9739) (50.6188, -96.0476) (50.6188, -95.1677) knots 0 0 0 1 2 2 2
  line L40 (50.6188, -95.1677) -> (50.6188, -92.075)
  spline S58 degree 2 poles (47.4232, -91.9669) (48.5656, -91.9669) (49.8212, -93.2483) (49.8212, -94.4318) knots 0 0 0 1 2 2 2
  spline S59 degree 2 poles (49.8212, -94.4318) (49.8212, -95.5948) (48.6016, -96.9739) (47.6188, -96.9739) knots 0 0 0 1 2 2 2
  spline S60 degree 2 poles (47.6188, -96.9739) (47.1762, -96.9739) (46.4918, -96.7166) (46.2397, -96.4438) knots 0 0 0 1 2 2 2
  spline S61 degree 2 poles (46.2397, -96.4438) (45.9824, -96.1711) (45.7097, -95.3838) (45.7097, -94.8126) knots 0 0 0 1 2 2 2
  line L41 (45.7097, -94.8126) -> (45.7097, -94.3752)
  line L42 (45.7097, -94.3752) -> (49.0082, -94.3752)
  spline S62 degree 2 poles (49.0082, -94.3752) (49.0082, -93.5467) (48.1745, -92.6668) (47.4335, -92.6668) knots 0 0 0 1 2 2 2
  spline S63 degree 2 poles (47.4335, -92.6668) (47.1711, -92.6668) (46.6616, -92.7851) (46.4558, -92.8778) knots 0 0 0 1 2 2 2
  spline S64 degree 2 poles (46.4558, -92.8778) (46.2397, -92.9807) (45.9412, -93.1608) (45.8434, -93.2431) knots 0 0 0 1 2 2 2
  line L43 (45.8434, -93.2431) -> (45.7971, -93.2431)
  line L44 (45.7971, -93.2431) -> (45.7971, -92.3683)
  spline S65 degree 2 poles (45.7971, -92.3683) (45.9361, -92.3117) (46.358, -92.147) (46.5227, -92.1007) knots 0 0 0 1 2 2 2
  spline S66 degree 2 poles (46.5227, -92.1007) (46.7543, -92.0338) (47.1351, -91.9669) (47.4232, -91.9669) knots 0 0 0 1 2 2 2
  spline S67 degree 2 poles (46.4918, -94.9876) (46.5021, -95.3118) (46.6359, -95.7852) (46.7646, -95.9447) knots 0 0 0 1 2 2 2
  spline S68 degree 2 poles (46.7646, -95.9447) (46.9035, -96.1248) (47.3409, -96.3152) (47.6651, -96.3152) knots 0 0 0 1 2 2 2
  spline S69 degree 2 poles (47.6651, -96.3152) (47.9841, -96.3152) (48.4318, -96.1248) (48.6171, -95.9395) knots 0 0 0 1 2 2 2
  spline S70 degree 2 poles (48.6171, -95.9395) (48.7972, -95.7491) (48.9824, -95.2912) (49.0082, -94.9876) knots 0 0 0 1 2 2 2
  line L45 (49.0082, -94.9876) -> (46.4918, -94.9876)
  line L46 (41.2328, -92.075) -> (42.0355, -92.075)
  line L47 (42.0355, -92.075) -> (42.0355, -92.5587)
  spline S71 degree 2 poles (42.0355, -92.5587) (42.2208, -92.4043) (42.4935, -92.1985) (42.6787, -92.111) knots 0 0 0 1 2 2 2
  spline S72 degree 2 poles (42.6787, -92.111) (42.8486, -92.0287) (43.2139, -91.9412) (43.4558, -91.9412) knots 0 0 0 1 2 2 2
  spline S73 degree 2 poles (43.4558, -91.9412) (43.8469, -91.9412) (44.5055, -92.2654) (44.7371, -92.5793) knots 0 0 0 1 2 2 2
  spline S74 degree 2 poles (44.7371, -92.5793) (44.9687, -92.8932) (45.2259, -93.8194) (45.2259, -94.4215) knots 0 0 0 1 2 2 2
  spline S75 degree 2 poles (45.2259, -94.4215) (45.2259, -95.0493) (44.9018, -95.9653) (44.6187, -96.31) knots 0 0 0 1 2 2 2
  spline S76 degree 2 poles (44.6187, -96.31) (44.3563, -96.6188) (43.6204, -96.9739) (43.2139, -96.9739) knots 0 0 0 1 2 2 2
  spline S77 degree 2 poles (43.2139, -96.9739) (42.8588, -96.9739) (42.3288, -96.8143) (42.0355, -96.6497) knots 0 0 0 1 2 2 2
  line L48 (42.0355, -96.6497) -> (42.0355, -98.708)
  line L49 (42.0355, -98.708) -> (41.2328, -98.708)
  line L50 (41.2328, -98.708) -> (41.2328, -92.075)
  line L51 (42.0355, -93.2328) -> (42.0355, -95.9859)
  spline S78 degree 2 poles (42.0355, -95.9859) (42.334, -96.1299) (42.8074, -96.238) (43.0801, -96.238) knots 0 0 0 1 2 2 2
  spline S79 degree 2 poles (43.0801, -96.238) (43.6976, -96.238) (44.3975, -95.3118) (44.3975, -94.437) knots 0 0 0 1 2 2 2
  spline S80 degree 2 poles (44.3975, -94.437) (44.3975, -93.593) (43.8623, -92.7028) (43.2705, -92.7028) knots 0 0 0 1 2 2 2
  spline S81 degree 2 poles (43.2705, -92.7028) (42.9566, -92.7028) (42.3185, -92.991) (42.0355, -93.2328) knots 0 0 0 1 2 2 2
  spline S82 degree 2 poles (33.3493, -94.5347) (33.3493, -93.3666) (34.4814, -91.9412) (35.3356, -91.9412) knots 0 0 0 1 2 2 2
  spline S83 degree 2 poles (35.3356, -91.9412) (35.7215, -91.9412) (36.2721, -92.1316) (36.5397, -92.2963) knots 0 0 0 1 2 2 2
  line L52 (36.5397, -92.2963) -> (36.5912, -92.075)
  line L53 (36.5912, -92.075) -> (37.3425, -92.075)
  line L54 (37.3425, -92.075) -> (37.3425, -98.708)
  line L55 (37.3425, -98.708) -> (36.5397, -98.708)
  line L56 (36.5397, -98.708) -> (36.5397, -96.3409)
  spline S84 degree 2 poles (36.5397, -96.3409) (36.2361, -96.6137) (35.5311, -96.9739) (35.0834, -96.9739) knots 0 0 0 1 2 2 2
  spline S85 degree 2 poles (35.0834, -96.9739) (34.2755, -96.9739) (33.3493, -95.6823) (33.3493, -94.5347) knots 0 0 0 1 2 2 2
  spline S86 degree 2 poles (34.1778, -94.473) (34.1778, -95.3272) (34.6975, -96.2123) (35.2738, -96.2123) knots 0 0 0 1 2 2 2
  spline S87 degree 2 poles (35.2738, -96.2123) (35.598, -96.2123) (36.267, -95.9035) (36.5397, -95.6668) knots 0 0 0 1 2 2 2
  line L57 (36.5397, -95.6668) -> (36.5397, -92.9344)
  spline S88 degree 2 poles (36.5397, -92.9344) (36.2361, -92.7851) (35.7678, -92.6616) (35.49, -92.6616) knots 0 0 0 1 2 2 2
  spline S89 degree 2 poles (35.49, -92.6616) (34.8776, -92.6616) (34.1778, -93.5313) (34.1778, -94.473) knots 0 0 0 1 2 2 2
  line L58 (28.7746, -96.8401) -> (31.3372, -90.3203)
  line L59 (31.3372, -90.3203) -> (32.1966, -90.3203)
  line L60 (32.1966, -90.3203) -> (31.3424, -92.3066)
  line L61 (31.3424, -92.3066) -> (33.0714, -96.8401)
  line L62 (33.0714, -96.8401) -> (32.2069, -96.8401)
  line L63 (32.2069, -96.8401) -> (30.905, -93.31)
  line L64 (30.905, -93.31) -> (29.6082, -96.8401)
  line L65 (29.6082, -96.8401) -> (28.7746, -96.8401)
  line L66 (67.5461, -81.4396) -> (68.6422, -81.4396)
  line L67 (68.6422, -81.4396) -> (70.6491, -83.9663)
  line L68 (70.6491, -83.9663) -> (71.6165, -83.9663)
  line L69 (71.6165, -83.9663) -> (71.6165, -81.4396)
  line L70 (71.6165, -81.4396) -> (72.4604, -81.4396)
  line L71 (72.4604, -81.4396) -> (72.4604, -87.7896)
  line L72 (72.4604, -87.7896) -> (70.8241, -87.7896)
  spline S90 degree 2 poles (70.8241, -87.7896) (70.2786, -87.7896) (69.5427, -87.6713) (69.2083, -87.4552) knots 0 0 0 1 2 2 2
  spline S91 degree 2 poles (69.2083, -87.4552) (68.8738, -87.239) (68.4878, -86.5649) (68.4878, -86.0658) knots 0 0 0 1 2 2 2
  spline S92 degree 2 poles (68.4878, -86.0658) (68.4878, -85.3711) (69.198, -84.4294) (69.8052, -84.203) knots 0 0 0 1 2 2 2
  line L73 (69.8052, -84.203) -> (67.5461, -81.4396)
  spline S93 degree 2 poles (69.3678, -85.9989) (69.3678, -86.2768) (69.5633, -86.7039) (69.7692, -86.8428) knots 0 0 0 1 2 2 2
  spline S94 degree 2 poles (69.7692, -86.8428) (69.9493, -86.9612) (70.4278, -87.0589) (70.7777, -87.0589) knots 0 0 0 1 2 2 2
  line L74 (70.7777, -87.0589) -> (71.6165, -87.0589)
  line L75 (71.6165, -87.0589) -> (71.6165, -84.6712)
  line L76 (71.6165, -84.6712) -> (70.8755, -84.6712)
  spline S95 degree 2 poles (70.8755, -84.6712) (70.5102, -84.6712) (69.9287, -84.7999) (69.728, -85.0006) knots 0 0 0 1 2 2 2
  spline S96 degree 2 poles (69.728, -85.0006) (69.5427, -85.1755) (69.3678, -85.6695) (69.3678, -85.9989) knots 0 0 0 1 2 2 2
  spline S97 degree 2 poles (63.1876, -83.8222) (63.1876, -82.618) (64.3454, -81.3058) (65.3128, -81.3058) knots 0 0 0 1 2 2 2
  spline S98 degree 2 poles (65.3128, -81.3058) (66.306, -81.3058) (67.4432, -82.6592) (67.4432, -83.8222) knots 0 0 0 1 2 2 2
  spline S99 degree 2 poles (67.4432, -83.8222) (67.4432, -85.016) (66.27, -86.3385) (65.3128, -86.3385) knots 0 0 0 1 2 2 2
  spline S100 degree 2 poles (65.3128, -86.3385) (64.3454, -86.3385) (63.1876, -85.0212) (63.1876, -83.8222) knots 0 0 0 1 2 2 2
  spline S101 degree 2 poles (64.0161, -83.8222) (64.0161, -84.7484) (64.6902, -85.649) (65.3128, -85.649) knots 0 0 0 1 2 2 2
  spline S102 degree 2 poles (65.3128, -85.649) (65.9355, -85.649) (66.6147, -84.7484) (66.6147, -83.8222) knots 0 0 0 1 2 2 2
  spline S103 degree 2 poles (66.6147, -83.8222) (66.6147, -82.9216) (65.9355, -81.9954) (65.3128, -81.9954) knots 0 0 0 1 2 2 2
  spline S104 degree 2 poles (65.3128, -81.9954) (64.6953, -81.9954) (64.0161, -82.9062) (64.0161, -83.8222) knots 0 0 0 1 2 2 2
  spline S105 degree 2 poles (58.3711, -83.8994) (58.3711, -82.7313) (59.5032, -81.3058) (60.3574, -81.3058) knots 0 0 0 1 2 2 2
  spline S106 degree 2 poles (60.3574, -81.3058) (60.7433, -81.3058) (61.2939, -81.4962) (61.5615, -81.6609) knots 0 0 0 1 2 2 2
  line L77 (61.5615, -81.6609) -> (61.613, -81.4396)
  line L78 (61.613, -81.4396) -> (62.3643, -81.4396)
  line L79 (62.3643, -81.4396) -> (62.3643, -88.0727)
  line L80 (62.3643, -88.0727) -> (61.5615, -88.0727)
  line L81 (61.5615, -88.0727) -> (61.5615, -85.7056)
  spline S107 degree 2 poles (61.5615, -85.7056) (61.2579, -85.9783) (60.5529, -86.3385) (60.1052, -86.3385) knots 0 0 0 1 2 2 2
  spline S108 degree 2 poles (60.1052, -86.3385) (59.2973, -86.3385) (58.3711, -85.0469) (58.3711, -83.8994) knots 0 0 0 1 2 2 2
  spline S109 degree 2 poles (59.1995, -83.8376) (59.1995, -84.6918) (59.7193, -85.5769) (60.2956, -85.5769) knots 0 0 0 1 2 2 2
  spline S110 degree 2 poles (60.2956, -85.5769) (60.6198, -85.5769) (61.2888, -85.2682) (61.5615, -85.0315) knots 0 0 0 1 2 2 2
  line L82 (61.5615, -85.0315) -> (61.5615, -82.299)
  spline S111 degree 2 poles (61.5615, -82.299) (61.2579, -82.1498) (60.7896, -82.0263) (60.5117, -82.0263) knots 0 0 0 1 2 2 2
  spline S112 degree 2 poles (60.5117, -82.0263) (59.8994, -82.0263) (59.1995, -82.8959) (59.1995, -83.8376) knots 0 0 0 1 2 2 2
  spline S113 degree 2 poles (52.9782, -81.3264) (53.6677, -81.3264) (54.6352, -81.6146) (55.0623, -81.8204) knots 0 0 0 1 2 2 2
  line L83 (55.0623, -81.8204) -> (55.0623, -82.8805)
  line L84 (55.0623, -82.8805) -> (55.0005, -82.8805)
  spline S114 degree 2 poles (55.0005, -82.8805) (54.5837, -82.4894) (53.5288, -82.0571) (53.0399, -82.0571) knots 0 0 0 1 2 2 2
  spline S115 degree 2 poles (53.0399, -82.0571) (52.3401, -82.0571) (51.6248, -82.6386) (51.6248, -83.1172) knots 0 0 0 1 2 2 2
  spline S116 degree 2 poles (51.6248, -83.1172) (51.6248, -83.498) (52.0005, -83.9714) (52.407, -84.0898) knots 0 0 0 1 2 2 2
  spline S117 degree 2 poles (52.407, -84.0898) (52.7003, -84.1721) (53.1892, -84.2853) (53.5545, -84.3779) knots 0 0 0 1 2 2 2
  spline S118 degree 2 poles (53.5545, -84.3779) (53.8839, -84.4654) (54.4036, -84.7278) (54.6043, -84.9388) knots 0 0 0 1 2 2 2
  spline S119 degree 2 poles (54.6043, -84.9388) (54.7998, -85.1498) (55.016, -85.7159) (55.016, -86.0864) knots 0 0 0 1 2 2 2
  spline S120 degree 2 poles (55.016, -86.0864) (55.016, -86.8582) (53.8118, -87.9028) (52.8804, -87.9028) knots 0 0 0 1 2 2 2
  spline S121 degree 2 poles (52.8804, -87.9028) (52.3453, -87.9028) (51.3984, -87.6919) (50.9919, -87.4912) knots 0 0 0 1 2 2 2
  line L85 (50.9919, -87.4912) -> (50.9919, -86.4826)
  line L86 (50.9919, -86.4826) -> (51.0536, -86.4826)
  spline S122 degree 2 poles (51.0536, -86.4826) (51.3572, -86.7605) (52.3041, -87.1721) (52.8238, -87.1721) knots 0 0 0 1 2 2 2
  spline S123 degree 2 poles (52.8238, -87.1721) (53.4104, -87.1721) (54.136, -86.6215) (54.136, -86.1738) knots 0 0 0 1 2 2 2
  spline S124 degree 2 poles (54.136, -86.1738) (54.136, -85.7725) (53.7089, -85.2939) (53.3075, -85.1858) knots 0 0 0 1 2 2 2
  spline S125 degree 2 poles (53.3075, -85.1858) (53.0399, -85.1138) (52.2629, -84.9285) (52.0056, -84.8513) knots 0 0 0 1 2 2 2
  spline S126 degree 2 poles (52.0056, -84.8513) (51.3521, -84.6507) (50.7449, -83.8428) (50.7449, -83.251) knots 0 0 0 1 2 2 2
  spline S127 degree 2 poles (50.7449, -83.251) (50.7449, -82.8753) (51.0485, -82.1549) (51.3212, -81.9028) knots 0 0 0 1 2 2 2
  spline S128 degree 2 poles (51.3212, -81.9028) (51.6248, -81.6249) (52.3967, -81.3264) (52.9782, -81.3264) knots 0 0 0 1 2 2 2
  spline S129 degree 2 poles (48.5064, -81.347) (49.16, -81.347) (49.8958, -82.0932) (49.8958, -82.9011) knots 0 0 0 1 2 2 2
  line L87 (49.8958, -82.9011) -> (49.8958, -85.5409)
  line L88 (49.8958, -85.5409) -> (50.4361, -85.5409)
  line L89 (50.4361, -85.5409) -> (50.4361, -86.2047)
  line L90 (50.4361, -86.2047) -> (49.8958, -86.2047)
  line L91 (49.8958, -86.2047) -> (49.8958, -87.5735)
  line L92 (49.8958, -87.5735) -> (49.0931, -87.5735)
  line L93 (49.0931, -87.5735) -> (49.0931, -86.2047)
  line L94 (49.0931, -86.2047) -> (47.6162, -86.2047)
  line L95 (47.6162, -86.2047) -> (47.6162, -85.5409)
  line L96 (47.6162, -85.5409) -> (49.0931, -85.5409)
  line L97 (49.0931, -85.5409) -> (49.0931, -83.2716)
  spline S130 degree 2 poles (49.0931, -83.2716) (49.0931, -82.9114) (49.0673, -82.5151) (48.9799, -82.3453) knots 0 0 0 1 2 2 2
  spline S131 degree 2 poles (48.9799, -82.3453) (48.9078, -82.1961) (48.5836, -82.0469) (48.3057, -82.0469) knots 0 0 0 1 2 2 2
  spline S132 degree 2 poles (48.3057, -82.0469) (48.1102, -82.0469) (47.7448, -82.1652) (47.6625, -82.2012) knots 0 0 0 1 2 2 2
  line L98 (47.6625, -82.2012) -> (47.6162, -82.2012)
  line L99 (47.6162, -82.2012) -> (47.6162, -81.4808)
  spline S133 degree 2 poles (47.6162, -81.4808) (47.8426, -81.4191) (48.3057, -81.347) (48.5064, -81.347) knots 0 0 0 1 2 2 2
  spline S134 degree 2 poles (44.9558, -81.3316) (46.0982, -81.3316) (47.3538, -82.6129) (47.3538, -83.7964) knots 0 0 0 1 2 2 2
  spline S135 degree 2 poles (47.3538, -83.7964) (47.3538, -84.9594) (46.1342, -86.3385) (45.1513, -86.3385) knots 0 0 0 1 2 2 2
  spline S136 degree 2 poles (45.1513, -86.3385) (44.7088, -86.3385) (44.0244, -86.0812) (43.7722, -85.8085) knots 0 0 0 1 2 2 2
  spline S137 degree 2 poles (43.7722, -85.8085) (43.5149, -85.5357) (43.2422, -84.7484) (43.2422, -84.1772) knots 0 0 0 1 2 2 2
  line L100 (43.2422, -84.1772) -> (43.2422, -83.7398)
  line L101 (43.2422, -83.7398) -> (46.5407, -83.7398)
  spline S138 degree 2 poles (46.5407, -83.7398) (46.5407, -82.9114) (45.7071, -82.0314) (44.9661, -82.0314) knots 0 0 0 1 2 2 2
  spline S139 degree 2 poles (44.9661, -82.0314) (44.7036, -82.0314) (44.1942, -82.1498) (43.9884, -82.2424) knots 0 0 0 1 2 2 2
  spline S140 degree 2 poles (43.9884, -82.2424) (43.7722, -82.3453) (43.4738, -82.5254) (43.376, -82.6078) knots 0 0 0 1 2 2 2
  line L102 (43.376, -82.6078) -> (43.3297, -82.6078)
  line L103 (43.3297, -82.6078) -> (43.3297, -81.733)
  spline S141 degree 2 poles (43.3297, -81.733) (43.4686, -81.6763) (43.8906, -81.5117) (44.0553, -81.4654) knots 0 0 0 1 2 2 2
  spline S142 degree 2 poles (44.0553, -81.4654) (44.2868, -81.3985) (44.6676, -81.3316) (44.9558, -81.3316) knots 0 0 0 1 2 2 2
  spline S143 degree 2 poles (44.0244, -84.3522) (44.0347, -84.6764) (44.1685, -85.1498) (44.2971, -85.3093) knots 0 0 0 1 2 2 2
  spline S144 degree 2 poles (44.2971, -85.3093) (44.4361, -85.4894) (44.8735, -85.6798) (45.1976, -85.6798) knots 0 0 0 1 2 2 2
  spline S145 degree 2 poles (45.1976, -85.6798) (45.5167, -85.6798) (45.9644, -85.4894) (46.1496, -85.3042) knots 0 0 0 1 2 2 2
  spline S146 degree 2 poles (46.1496, -85.3042) (46.3297, -85.1138) (46.515, -84.6558) (46.5407, -84.3522) knots 0 0 0 1 2 2 2
  line L104 (46.5407, -84.3522) -> (44.0244, -84.3522)
  spline S147 degree 2 poles (40.3605, -81.3316) (41.5029, -81.3316) (42.7585, -82.6129) (42.7585, -83.7964) knots 0 0 0 1 2 2 2
  spline S148 degree 2 poles (42.7585, -83.7964) (42.7585, -84.9594) (41.5389, -86.3385) (40.5561, -86.3385) knots 0 0 0 1 2 2 2
  spline S149 degree 2 poles (40.5561, -86.3385) (40.1135, -86.3385) (39.4291, -86.0812) (39.177, -85.8085) knots 0 0 0 1 2 2 2
  spline S150 degree 2 poles (39.177, -85.8085) (38.9197, -85.5357) (38.647, -84.7484) (38.647, -84.1772) knots 0 0 0 1 2 2 2
  line L105 (38.647, -84.1772) -> (38.647, -83.7398)
  line L106 (38.647, -83.7398) -> (41.9455, -83.7398)
  spline S151 degree 2 poles (41.9455, -83.7398) (41.9455, -82.9114) (41.1118, -82.0314) (40.3708, -82.0314) knots 0 0 0 1 2 2 2
  spline S152 degree 2 poles (40.3708, -82.0314) (40.1084, -82.0314) (39.5989, -82.1498) (39.3931, -82.2424) knots 0 0 0 1 2 2 2
  spline S153 degree 2 poles (39.3931, -82.2424) (39.177, -82.3453) (38.8785, -82.5254) (38.7807, -82.6078) knots 0 0 0 1 2 2 2
  line L107 (38.7807, -82.6078) -> (38.7344, -82.6078)
  line L108 (38.7344, -82.6078) -> (38.7344, -81.733)
  spline S154 degree 2 poles (38.7344, -81.733) (38.8734, -81.6763) (39.2953, -81.5117) (39.46, -81.4654) knots 0 0 0 1 2 2 2
  spline S155 degree 2 poles (39.46, -81.4654) (39.6916, -81.3985) (40.0724, -81.3316) (40.3605, -81.3316) knots 0 0 0 1 2 2 2
  spline S156 degree 2 poles (39.4291, -84.3522) (39.4394, -84.6764) (39.5732, -85.1498) (39.7019, -85.3093) knots 0 0 0 1 2 2 2
  spline S157 degree 2 poles (39.7019, -85.3093) (39.8408, -85.4894) (40.2782, -85.6798) (40.6024, -85.6798) knots 0 0 0 1 2 2 2
  spline S158 degree 2 poles (40.6024, -85.6798) (40.9214, -85.6798) (41.3691, -85.4894) (41.5544, -85.3042) knots 0 0 0 1 2 2 2
  spline S159 degree 2 poles (41.5544, -85.3042) (41.7345, -85.1138) (41.9197, -84.6558) (41.9455, -84.3522) knots 0 0 0 1 2 2 2
  line L109 (41.9455, -84.3522) -> (39.4291, -84.3522)
  line L110 (37.0157, -81.4396) -> (37.8185, -81.4396)
  line L111 (37.8185, -81.4396) -> (37.8185, -88.0727)